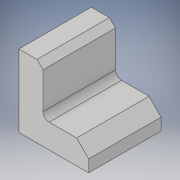
# Autodesk Inventor part: ChamferAngle
Saved by Autodesk Inventor 2018 (Build 220112000, 112)
## iProperties
Created: 2019-01-09
Part Number: ChamferAngle
Material: Generic
Document SubType Name: Modeling
Designer: 10043883
Density: 1 g/cm^3
Appearance: Default
Author: 10043883
Autodesk Inventor part; units mm, degrees
ref_plane "YZ Plane" through (0, 0, 0) normal (1, 0, 0) x (0, 1, 0)
ref_plane "XZ Plane" through (0, 0, 0) normal (0, 1, 0) x (-1, 0, 0)
ref_plane "XY Plane" through (0, 0, 0) normal (0, 0, 1) x (1, 0, 0)
sketch "Sketch1" plane through (0, 0, 0) normal (0, 0, 1) x (1, 0, 0)
  line L0 (-15.2972, 20.3009) -> (-2.5972, 20.3009)
  line L1 (-2.5972, 20.3009) -> (-2.5972, -5.0991)
  line L2 (-1.0722, -17.7991) -> (-15.2972, -17.7991)
  line L3 (-15.2972, -17.7991) -> (-15.2972, 20.3009)
  line L4 (-2.5972, -5.0991) -> (21.4362, -5.0991)
  line L5 (21.4362, -5.0991) -> (21.4362, -17.7991)
  line L6 (21.4362, -17.7991) -> (-1.0722, -17.7991)
  point P0 (0, 0)
  dimension "d0" = 38.1
  dimension "d1" = 12.7
  dimension "d2" = 25.4
  constraints: 14 end point, 3 parallel, 2 horizontal, 2 perpendicular
  measures "d0" distance of L2.end L0.start
  measures "d1" distance of L0.start L0.end
  measures "d2" distance of L0.end L1.end
extrude "Extrusion1" add sketch "Sketch1" along normal blind 38.1
chamfer "Chamfer1" distance 3.175 angle 45 1 edges at (-2.5972, 20.3009, 19.05)
chamfer "Chamfer2" distance 6.35 angle 45 1 edges at (21.4362, -5.0991, 19.05)
fillet "Fillet2" radius 3.175 1 edges at (-2.5972, -5.0991, 19.05)
body "Solid1"
